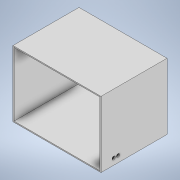
# Autodesk Inventor part: mouse_SP_box
Saved by Autodesk Inventor 2020 (Build 240168000, 168)
## iProperties
Created: 2019-06-13
Part Number: mouse_SP_box
Material: Generic
Document SubType Name: Modeling
Designer: Dammy
Density: 1 g/cm^3
Appearance: Default
Author: Dammy
Autodesk Inventor part; units mm, degrees
ref_plane "YZ Plane" through (0, 0, 0) normal (1, 0, 0) x (0, 1, 0)
ref_plane "XZ Plane" through (0, 0, 0) normal (0, 1, 0) x (-1, 0, 0)
ref_plane "XY Plane" through (0, 0, 0) normal (0, 0, 1) x (1, 0, 0)
sketch "Sketch2" plane through (0, 0, 0) normal (0, 0, 1) x (1, 0, 0)
  line L0 (200, -150) -> (-200, -150)
  line L1 (-200, -150) -> (-200, 150)
  line L2 (-200, 150) -> (200, 150)
  line L3 (200, 150) -> (200, -150)
  line L4 (200, -150) -> (-200, 150) construction
  line L5 (-200, -150) -> (200, 150) construction
  point P0 (0, 0)
  dimension "d0" = 400
  dimension "d1" = 300
  constraints: 12 end point, 2 midpoint, 2 parallel, 1 horizontal, 1 perpendicular
  measures "d0" distance of L1.end L2.end
  measures "d1" distance of L0.end L1.end
extrude "Base" add sketch "Sketch2" along normal blind 300
shell "Shell1" thickness 5 removed faces 1 at (66.6667, -50, 300)
sketch "Sketch3" plane through (0, 0, 0) normal (0, 0, -1) x (-1, 0, 0)
  circle A0 centre (-167.85, 85.85) radius 2.15
  line L0 (-200, 150) -> (200, 150) construction
  line L1 (-200, 150) -> (200, 150) construction
  line L2 (200, 150) -> (200, -150) construction
  line L3 (200, -150) -> (-200, -150) construction
  line L4 (-200, -150) -> (-200, 150) construction
  circle A1 centre (-135.85, 85.85) radius 2.15
  circle A2 centre (-167.85, 117.85) radius 2.15
  circle A3 centre (-135.85, 117.85) radius 2.15
  point P0 (0, 0)
  dimension "d5" = 4.3
  dimension "d8" = 32
  dimension "d11" = 32
  dimension "d14" = 32.15
  dimension "d15" = 32.15
  constraints: 8 end point, 4 centre point, 2 horizontal, 2 parallel, 1 perpendicular, 1 vertical, 6 other
  measures "d5" diameter of A0
  measures "d8" distance of A0.centre A1.centre
  measures "d11" distance of A0.centre A2.centre
  measures "d14" distance from line of L0 A2.centre
  measures "d15" distance from line of L4 A2.centre
extrude "40 mm fan mout holes" cut sketch "Sketch3" against normal up to surface (5 mm away)
sketch "Sketch4" plane through (200, -150, 0) normal (1, 0, 0) x (0, 0, -1)
  circle A0 centre (-242.5, 28.75) radius 7.5
  line L0 (-300, 0) -> (-300, 300) projected
  line L1 (0, 0) -> (-300, 0) projected
  circle A1 centre (-222.5, 28.75) radius 7.5
  point P0 (0, 150)
  dimension "d18" = 15
  dimension "d19" = 57.5
  dimension "d20" = 28.75
  dimension "d23" = 20
  constraints: 2 centre point, 1 horizontal, 2 other
  measures "d18" diameter of A0
  measures "d19" distance from line of L0 A0.centre
  measures "d20" distance from line of L1 A0.centre
  measures "d23" distance of A0.centre A1.centre
extrude "Cable Holes" cut sketch "Sketch4" against normal up to surface (5 mm away)
equation "\"d15\" = d14"
equation "\"d20\" = 0.5 * d19"
body "Solid1"
